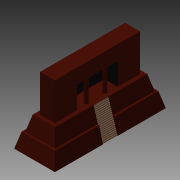
# Autodesk Inventor part: Side1
Saved by Autodesk Inventor 2015 (Build 190159000, 159)
## iProperties
Created: 2016-12-01
Part Number: Side1
Material: Generic
Document SubType Name: Modeling
Designer: Simms
Density: 1 g/cm^3
Appearance: Default
Author: Simms
Autodesk Inventor part; units mm, degrees
sketch "Sketch1" plane through (0, 0, 0) normal (0, 1, 0) x (-1, 0, 0)
  line L0 (0, 0) -> (69.85, 0)
  line L1 (69.85, 0) -> (69.85, -190.5)
  line L2 (69.85, -190.5) -> (0, -190.5)
  line L3 (0, -190.5) -> (0, 0)
  dimension "d0" = 69.85
  dimension "d1" = 190.5
  constraints: 8 end point, 2 parallel, 1 horizontal, 1 perpendicular
  measures "d0" distance of L1.end L2.end
  measures "d1" distance of L0.end L1.end
ref_plane "Work Plane1" through (0, 25.4, 0) normal (0, 1, 0) x (-1, 0, 0)
sketch "Sketch2" plane through (0, 25.4, 0) normal (0, 1, 0) x (-1, 0, 0)
  line L0 (0, 0) -> (69.85, 0) projected
  line L1 (69.85, -190.5) -> (0, -190.5) projected
  line L2 (69.85, 0) -> (69.85, -190.5) projected
  line L3 (0, -190.5) -> (0, 0) projected
  line L4 (63.5, -184.15) -> (6.35, -184.15)
  line L5 (6.35, -184.15) -> (6.35, -6.35)
  line L6 (6.35, -6.35) -> (63.5, -6.35)
  line L7 (63.5, -6.35) -> (63.5, -184.15)
  dimension "d3" = 6.35
  constraints: 8 end point, 3 other
  measures "d3" distance between parallel lines of L2 L7
loft "Loft1" add profiles "Sketch1", "Sketch2" contours all / L4 L5 L6 L7
sketch "Sketch3" plane through (-63.5, 25.4, -6.35) normal (0, 1, 0) x (1, 0, 0)
  line L0 (57.15, 0) -> (0, 0) projected
  line L1 (57.15, 177.8) -> (57.15, 0) projected
  line L2 (0, 177.8) -> (57.15, 177.8) projected
  line L3 (0, 0) -> (0, 177.8) projected
  line L4 (3.175, 174.625) -> (53.975, 174.625)
  line L5 (53.975, 174.625) -> (53.975, 3.175)
  line L6 (53.975, 3.175) -> (3.175, 3.175)
  line L7 (3.175, 3.175) -> (3.175, 174.625)
  point P0 (63.5, -6.35)
  dimension "d8" = 3.175
  constraints: 8 end point, 3 other
  measures "d8" distance between parallel lines of L3 L7
ref_plane "Work Plane2" through (-63.5, 50.8, -6.35) normal (0, 1, 0) x (1, 0, 0)
sketch "Sketch4" plane through (-63.5, 50.8, -6.35) normal (0, 1, 0) x (1, 0, 0)
  line L0 (53.975, 3.175) -> (3.175, 3.175) projected
  line L1 (3.175, 3.175) -> (3.175, 174.625) projected
  line L2 (53.975, 174.625) -> (53.975, 3.175) projected
  line L3 (3.175, 174.625) -> (53.975, 174.625) projected
  line L4 (9.525, 168.275) -> (9.525, 9.525)
  line L5 (9.525, 9.525) -> (47.625, 9.525)
  line L6 (47.625, 9.525) -> (47.625, 168.275)
  line L7 (47.625, 168.275) -> (9.525, 168.275)
  point P0 (63.5, -6.35)
  dimension "d10" = 6.35
  constraints: 8 end point, 3 other
  measures "d10" distance between parallel lines of L1 L4
loft "Loft2" add profiles "Sketch3", "Sketch4" contours L4 L5 L6 L7 / L7 L6 L5 L4
sketch "Sketch5" plane through (-53.975, 50.8, -174.625) normal (0, 1, 0) x (1, 0, 0)
  line L0 (0, 0) -> (38.1, 0) projected
  line L1 (0, -158.75) -> (0, 0) projected
  line L2 (38.1, -158.75) -> (0, -158.75) projected
  line L3 (38.1, 0) -> (38.1, -158.75) projected
  line L4 (6.35, -6.35) -> (31.75, -6.35)
  line L5 (31.75, -152.4) -> (6.35, -152.4)
  line L6 (31.75, -114.3) -> (8.89, -114.3)
  line L7 (31.75, -44.45) -> (8.89, -44.45)
  line L8 (6.35, -152.4) -> (6.35, -114.3)
  line L9 (6.35, -44.45) -> (6.35, -6.35)
  line L10 (31.75, -6.35) -> (31.75, -44.45)
  line L11 (31.75, -114.3) -> (31.75, -152.4)
  line L12 (6.35, -44.45) -> (6.35, -114.3)
  line L13 (8.89, -114.3) -> (8.89, -44.45)
  circle A0 centre (28.575, -95.25) radius 3.175
  circle A1 centre (28.575, -63.5) radius 3.175
  point P0 (53.975, -174.625)
  dimension "d16" = 146.05
  dimension "d17" = 38.1
  dimension "d19" = 38.1
  dimension "d20" = 2.54
  dimension "d21" = 6.35
  dimension "d22" = 6.35
  dimension "d23" = 19.05
  dimension "d24" = 19.05
  dimension "d25" = 3.175
  dimension "d26" = 3.175
  constraints: 20 end point, 5 perpendicular, 2 centre point, 2 vertical, 1 collinear
  measures "d16" distance between parallel lines of L4 L5
  measures "d17" distance between parallel lines of L5 L6
  measures "d19" distance between parallel lines of L4 L7
  measures "d20" distance between parallel lines of L13 L12
  measures "d21" diameter of A0
  measures "d22" diameter of A1
  measures "d23" distance from line of A1.centre L7
  measures "d24" distance from line of A0.centre L6
  measures "d25" distance from line of A0.centre L11
  measures "d26" distance from line of A1.centre L10
extrude "Extrusion1" add sketch "Sketch5" along normal blind 38.1 contours L4 L10 L7 L13 L6 L11 L5 L8 L12 L9 | A0 | A1
sketch "Sketch6" plane through (-53.975, 88.9, -174.625) normal (0, 1, 0) x (1, 0, 0)
  line L0 (6.35, -6.35) -> (31.75, -6.35)
  line L1 (31.75, -6.35) -> (31.75, -152.4)
  line L2 (31.75, -152.4) -> (6.35, -152.4)
  line L3 (6.35, -152.4) -> (6.35, -6.35)
  line L4 (6.35, -152.4) -> (31.75, -152.4) projected
  point P0 (53.975, -174.625)
  constraints: 8 end point, 2 parallel, 1 horizontal, 1 perpendicular, 1 point on line
extrude "Extrusion2" add sketch "Sketch6" along normal blind 25.4
ref_plane "Work Plane3" through (-47.625, 50.8, -95.25) normal (0, 0, 1) x (1, 0, 0)
sketch "Sketch7" plane through (-47.625, 50.8, -95.25) normal (0, 0, 1) x (1, 0, 0)
  line L0 (31.75, 0) -> (31.75, -50.8)
  line L1 (31.75, -50.8) -> (47.625, -50.8)
  line L2 (47.625, -50.8) -> (38.6676, 0)
  line L3 (38.6676, 0) -> (31.75, 0)
  dimension "d31" = 80
  constraints: 8 end point, 1 perpendicular, 1 point on line, 1 vertical
  measures "d31" angle of L2 L1
extrude "Extrusion3" add sketch "Sketch7" along normal mid plane 25.4
sketch "Sketch8" plane through (-47.625, 50.8, -82.55) normal (0, 0, 1) x (1, 0, 0)
  line L0 (31.75, 0) -> (31.75, -2.54)
  line L1 (38.6676, 0) -> (31.75, 0) projected
  line L2 (31.75, 0) -> (34.29, 0) construction
  line L3 (31.75, -2.54) -> (33.02, -2.54)
  line L4 (31.75, 0) -> (31.75, 27.4808)
  line L5 (31.75, 27.4808) -> (33.02, 27.4808)
  line L6 (33.02, 27.4808) -> (33.02, -2.54)
  point P0 (47.625, -50.8)
  dimension "d34" = 2.54
  dimension "d35" = 270
  dimension "d36" = 1.27
  dimension "d37" = 90
  constraints: 12 end point, 5 perpendicular, 1 horizontal, 1 vertical
  measures "d34" distance of L0.start L0.end
  measures "d36" distance of L0.end L3.end
  measures "d37" angle of L3 L0
extrude "Extrusion4" cut sketch "Sketch8" against normal blind 25.4
pattern_linear "Rectangular Pattern1" count 20 spacing 2.667 along (0.2983, -0.9545, 0) of "Extrusion4"
body "Solid1"
